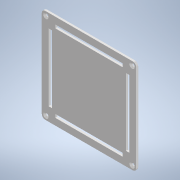
# Autodesk Inventor part: Led deksel niet hub
Saved by Autodesk Inventor 2021 (Build 250183000, 183)
## iProperties
Created: 2023-10-02
Part Number: Led deksel niet hub
Material: Generic
Document SubType Name: Modeling
Designer: Elias
Density: 1 g/cm^3
Appearance: Default
Author: Elias
Autodesk Inventor part; units mm, degrees
ref_plane "YZ Plane" through (0, 0, 0) normal (1, 0, 0) x (0, 1, 0)
ref_plane "XZ Plane" through (0, 0, 0) normal (0, 1, 0) x (-1, 0, 0)
ref_plane "XY Plane" through (0, 0, 0) normal (0, 0, 1) x (1, 0, 0)
sketch "Sketch1" plane through (0, 0, 0) normal (0, 0, 1) x (1, 0, 0)
  line L0 (0, 0) -> (140, 0)
  line L1 (140, 0) -> (140, 140)
  line L2 (140, 140) -> (0, 140)
  line L3 (0, 140) -> (0, 0)
  dimension "d0" = 140
  dimension "d1" = 140
  constraints: 8 end point, 2 parallel, 1 horizontal, 1 perpendicular
  measures "d0" distance of L1.end L2.end
  measures "d1" distance of L0.end L1.end
extrude "Extrusion1" add sketch "Sketch1" along normal blind 3
fillet "Fillet1" radius 5 4 edges at (140, 140, 1.5) (140, 0, 1.5) (0, 140, 1.5) (0, 0, 1.5)
sketch "Sketch4" plane through (0, 0, 3) normal (0, 0, 1) x (1, 0, 0)
  line L0 (135, 140) -> (5, 140) projected
  line L1 (0, 135) -> (0, 5) projected
  line L2 (140, 5) -> (140, 135) projected
  line L3 (5, 0) -> (135, 0) projected
  point P0 (0, 0)
  point P1 (6, 134)
  point P2 (134, 134)
  point P3 (6, 6)
  point P4 (134, 6)
  dimension "d30" = 6
  dimension "d31" = 6
  dimension "d32" = 6
  dimension "d33" = 6
  dimension "d34" = 6
  dimension "d35" = 6
  dimension "d36" = 6
  dimension "d37" = 6
  measures "d30" distance from line of L0 point (6, 134)
  measures "d31" distance from line of L1 point (6, 134)
  measures "d32" distance from line of L2 point (134, 134)
  measures "d33" distance from line of L0 point (134, 134)
  measures "d34" distance from line of L3 point (134, 6)
  measures "d35" distance from line of point (134, 6) L2
  measures "d36" distance from line of L1 point (6, 6)
  measures "d37" distance from line of L3 point (6, 6)
hole "Hole2" at (134, 134, 3) at (6, 6, 3) at (134, 6, 3) at (6, 134, 3) direction (0, 0, -1) diameter 4 depth 15
sketch "Sketch5" plane through (0, 0, 3) normal (0, 0, 1) x (1, 0, 0)
  line L0 (20, 130) -> (120, 130)
  line L1 (120, 130) -> (120, 125)
  line L2 (120, 125) -> (20, 125)
  line L3 (20, 125) -> (20, 130)
  line L4 (135, 140) -> (5, 140) projected
  line L5 (140, 5) -> (140, 135) projected
  line L6 (20, 15) -> (120, 15)
  line L7 (120, 15) -> (120, 10)
  line L8 (120, 10) -> (20, 10)
  line L9 (20, 10) -> (20, 15)
  line L10 (5, 0) -> (135, 0) projected
  line L11 (10, 120) -> (15, 120)
  line L12 (15, 120) -> (15, 20)
  line L13 (15, 20) -> (10, 20)
  line L14 (10, 20) -> (10, 120)
  line L15 (0, 135) -> (0, 5) projected
  line L16 (125, 120) -> (130, 120)
  line L17 (130, 120) -> (130, 20)
  line L18 (130, 20) -> (125, 20)
  line L19 (125, 20) -> (125, 120)
  point P0 (0, 0)
  dimension "d45" = 10
  dimension "d46" = 5
  dimension "d47" = 20
  dimension "d48" = 100
  dimension "d49" = 100
  dimension "d50" = 5
  dimension "d51" = 20
  dimension "d52" = 10
  dimension "d53" = 5
  dimension "d54" = 100
  dimension "d55" = 20
  dimension "d56" = 10
  dimension "d57" = 5
  dimension "d58" = 100
  dimension "d59" = 10
  dimension "d60" = 20
  constraints: 32 end point, 8 parallel, 4 horizontal, 4 perpendicular
  measures "d45" distance between parallel lines of L4 L0
  measures "d46" distance of L0.end L1.end
  measures "d47" distance between parallel lines of L5 L1
  measures "d48" distance of L0.start L0.end
  measures "d49" distance of L6.start L6.end
  measures "d50" distance of L6.end L7.end
  measures "d51" distance from line of L5 L6.end
  measures "d52" distance between parallel lines of L10 L8
  measures "d53" distance of L11.start L11.end
  measures "d54" distance of L11.end L12.end
  measures "d55" distance between parallel lines of L10 L13
  measures "d56" distance between parallel lines of L15 L14
  measures "d57" distance of L16.start L16.end
  measures "d58" distance of L16.end L17.end
  measures "d59" distance between parallel lines of L5 L17
  measures "d60" distance between parallel lines of L10 L18
extrude "Extrusion4" cut sketch "Sketch5" against normal blind 10
chamfer "Chamfer1" distance 2 angle 45 4 edges at (6, 136, 3) (134, 136, 3) (134, 8, 3) (6, 8, 3)
body "Solid1"
